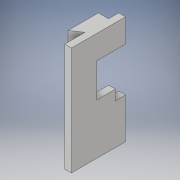
# Autodesk Inventor part: Inner Rails 2
Saved by Autodesk Inventor 2019 (Build 230136000, 136)
## iProperties
Created: 2019-03-02
Part Number: Inner Rails 2
Material: Generic
Document SubType Name: Modeling
Designer: Jared
Density: 1 g/cm^3
Appearance: Default
Author: Jared
Autodesk Inventor part; units mm, degrees
ref_plane "YZ Plane" through (0, 0, 0) normal (1, 0, 0) x (0, 1, 0)
ref_plane "XZ Plane" through (0, 0, 0) normal (0, 1, 0) x (-1, 0, 0)
ref_plane "XY Plane" through (0, 0, 0) normal (0, 0, 1) x (1, 0, 0)
sketch "Sketch1" plane through (0, 0, 0) normal (0, 1, 0) x (-1, 0, 0)
  line L0 (0, 0) -> (0, -16)
  line L1 (0, -16) -> (2, -16)
  line L2 (0, 0) -> (2, 0)
  line L3 (2, 0) -> (2, -6)
  line L4 (2, -16) -> (2, -13)
  line L5 (2, -13) -> (5, -13)
  line L6 (5, -13) -> (5, -4)
  line L7 (5, -4) -> (2, -6)
  dimension "d0" = 16
  dimension "d1" = 2
  dimension "d2" = 6
  dimension "d3" = 3
  dimension "d4" = 3
  dimension "d5" = 9
  constraints: 16 end point, 3 vertical, 2 parallel, 2 perpendicular, 1 horizontal
  measures "d0" distance of L0.start L0.end
  measures "d1" distance of L0.end L1.end
  measures "d2" distance of L2.end L3.end
  measures "d3" distance of L1.end L4.end
  measures "d4" distance of L4.end L5.end
  measures "d5" distance of L5.end L6.end
extrude "Extrusion1" add sketch "Sketch1" along normal blind 32
sketch "Sketch2" plane through (-5, 0, -13) normal (-1, 0, 0) x (0, 0, 1)
  line L0 (0, 0) -> (9, 0) projected
  line L1 (9, 0) -> (9, 32) projected
  line L2 (0, 32) -> (9, 32) projected
  line L3 (0, 0) -> (0, 32) projected
  line L4 (0, 0) -> (9, 0) projected
  line L5 (5.5, 0) -> (5.5, 25)
  line L6 (5.5, 25) -> (0, 25)
  point P0 (13, 0)
  dimension "d8" = 25
  dimension "d9" = 5.5
  constraints: 4 end point, 2 perpendicular, 2 point on line
  measures "d8" distance of L5.start L5.end
  measures "d9" distance of L5.end L6.end
extrude "Extrusion2" cut sketch "Sketch2" against normal blind 3 contours L3 L6 L5 L0
sketch "Sketch3" plane through (-2, 0, -16) normal (-1, 0, 0) x (0, 0, 1)
  line L0 (0, 0) -> (8.5, 0) projected
  line L1 (8.5, 25) -> (8.5, 0) projected
  line L2 (3, 25) -> (8.5, 25) projected
  line L3 (3, 25) -> (3, 32) projected
  line L4 (0, 32) -> (3, 32) projected
  line L5 (0, 0) -> (0, 32) projected
  line L6 (0, 0) -> (8.5, 0) projected
  line L7 (0, 0) -> (0, 12)
  line L8 (0, 0) -> (0, 32) projected
  line L9 (0, 12) -> (3, 12)
  line L10 (3, 12) -> (3, 15)
  line L11 (3, 15) -> (8.5, 15)
  line L12 (8.5, 25) -> (8.5, 0) projected
  line L13 (3, 25) -> (3, 32) projected
  line L14 (3, 25) -> (0, 25)
  point P0 (16, 0)
  dimension "d12" = 12
  dimension "d13" = 3
  dimension "d14" = 3
  constraints: 10 end point, 4 perpendicular, 3 point on line
  measures "d12" distance of L0.start L7.end
  measures "d13" distance of L7.end L9.end
  measures "d14" distance of L9.end L10.end
extrude "Extrusion3" cut sketch "Sketch3" against normal blind 4 contours L5 L14 L2 L1 L11 L10 L9
body "Solid1"
